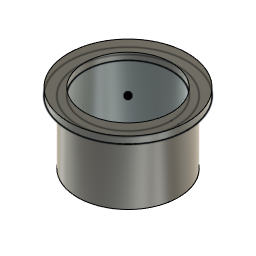
Turbine (Autodesk Fusion 360 archive; units mm, degrees)
design "turbine 5.0"
Autodesk Fusion 360 part; units mm, degrees
sketch "Sketch1" plane through (0, 0, 0) normal (0, 0, 1) x (1, 0, 0)
  circle A0 centre (0, 0) radius 61.85
  circle A1 centre (0, 0) radius 71.85
  circle A2 centre (0, 0) radius 84.85
  dimension "d1" = 123.7
  dimension "d2" = 10
  dimension "d3" = 169.7
  constraint coincident A0.centre A1.centre
  measures "d1" diameter of A0
  measures "d3" diameter of A2
extrude "Extrude1" add sketch "Sketch1" against normal blind 90 contours A1 makes body 1
extrude "Extrude2" add sketch "Sketch1" along normal blind 10 separate body contours A1 | A2 makes body 2

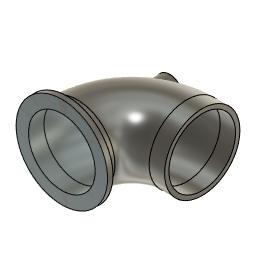
design "turbine 4"
Autodesk Fusion 360 part; units mm, degrees
sketch "Sketch1" plane through (0, 0, 0) normal (0, 1, 0) x (1, 0, 0)
  circle A0 centre (0, 0) radius 69.85
  line L0 (0, 0, 0) -> (0, 0, 28.6207)
  line L1 (101.6, 0, 130.2207) -> (130.2207, 0, 130.2207)
  arc A1 through (101.6, 0, 130.2207) (29.758, 0, 100.4627) (0, 0, 28.6207)
  circle A2 centre (0, 0) radius 61.85
  dimension "d1" = 139.7
  dimension "d2" = 101.6
  constraint coincident A0.centre A2.centre
  measures "d1" diameter of A0
sweep "Sweep1" add profiles "Sketch1" path "Sketch1" along L0 A1 L1 section 1
sketch "Sketch2" plane through (0, 0, 0) normal (0, 1, 0) x (1, 0, 0)
  circle A0 centre (0, 0) radius 69.85
  circle A1 centre (0, 0) radius 84.85
  circle A2 centre (0, 0) radius 7.5
  dimension "d10" = 15
  dimension "d13" = 15
  constraint coincident A0.centre A1.centre
  measures "d13" diameter of A2
extrude "Extrude1" add sketch "Sketch2" along normal blind 10 contours A1
extrude "Extrude2" cut sketch "Sketch2" along normal blind 270 contours A2
ref_plane "WorkPlane1" through (0, 200, 0) normal (0, -1, 0) x (0, 0, -1)
sketch "Sketch3" plane through (0, 0, 0) normal (0, -1, 0) x (1, 0, 0)
  circle A0 centre (0, 0) radius 84.85
  circle A1 centre (0, 0) radius 61.85
sketch "Sketch4" plane through (0, 200, 0) normal (0, -1, 0) x (1, 0, 0)
  circle A0 centre (0, 0) radius 25
  dimension "d17" = 50
  constraint coincident A0.centre origin
  measures "d17" diameter of A0
extrude "Extrude3" add sketch "Sketch4" along normal up to surface end surface at (21.5773, 170.1109, -10.5021)
sketch "Sketch5" plane through (0, 200, 0) normal (0, 1, 0) x (-1, 0, 0)
  circle A0 centre (0, 0) radius 25
  circle A1 centre (0, 0) radius 17.6
  dimension "d20" = 35.2
  constraint coincident A0.centre A1.centre
  measures "d20" diameter of A1
extrude "Extrude4" cut sketch "Sketch5" against normal blind 20 contours A1
sketch "Sketch6" plane through (0, 180, 0) normal (0, 1, 0) x (-1, 0, 0)
  circle A0 centre (0, 0) radius 17.6
  circle A1 centre (0, 0) radius 8.5
  dimension "d23" = 17
  constraint concentric A0 A1
  measures "d23" diameter of A1
extrude "Extrude5" cut sketch "Sketch6" against normal blind 310 contours A1
